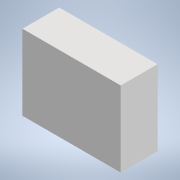
# Autodesk Inventor part: motor_controller_sketch
Saved by Autodesk Inventor 2020 (Build 240168000, 168)
## iProperties
Created: 2019-10-22
Part Number: motor_controller_sketch
Material: Generic
Document SubType Name: Modeling
Designer: Connor
Density: 1 g/cm^3
Appearance: Default
Author: Connor
Autodesk Inventor part; units mm, degrees
ref_plane "YZ Plane" through (0, 0, 0) normal (1, 0, 0) x (0, 1, 0)
ref_plane "XZ Plane" through (0, 0, 0) normal (0, 1, 0) x (-1, 0, 0)
ref_plane "XY Plane" through (0, 0, 0) normal (0, 0, 1) x (1, 0, 0)
sketch "Sketch1" plane through (0, 0, 0) normal (0, 0, 1) x (1, 0, 0)
  line L0 (0, 0) -> (0, 55.118)
  line L1 (0, 55.118) -> (71.882, 55.118)
  line L2 (71.882, 55.118) -> (71.882, 0)
  line L3 (71.882, 0) -> (0, 0)
  dimension "d0" = 55.118
  dimension "d1" = 71.882
  constraints: 8 end point, 3 perpendicular, 1 vertical
  measures "d0" distance of L0.start L0.end
  measures "d1" distance of L0.end L1.end
extrude "Extrusion1" add sketch "Sketch1" along normal blind 26.924
sketch "Sketch4" plane through (0, 0, 0) normal (-1, 0, 0) x (0, 0, 1)
  line L0 (5.7909, 6.9155) -> (5.7909, 47.856) construction
  line L1 (5.7909, 47.856) -> (8.0781, 47.856) construction
  line L2 (8.0781, 47.856) -> (8.0781, 6.9155) construction
  line L3 (8.0781, 6.9155) -> (5.7909, 6.9155) construction
  point P0 (0, 0)
  constraints: 2 other
body "Solid1"
